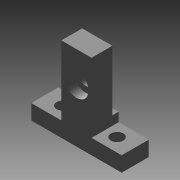
# Autodesk Inventor part: Linear Bearing Adapter Arm
Saved by Autodesk Inventor 2015 SP1 (Build 190203100, 203)
## iProperties
Created: 2015-05-06
Part Number: Linear Bearing Adapter Arm
Material: Generic
Document SubType Name: Modeling
Designer: Andrew
Density: 1 g/cm^3
Appearance: Default
Author: Andrew
Autodesk Inventor part; units mm, degrees
ref_plane "YZ Plane" through (0, 0, 0) normal (1, 0, 0) x (0, 1, 0)
ref_plane "XZ Plane" through (0, 0, 0) normal (0, 1, 0) x (-1, 0, 0)
ref_plane "XY Plane" through (0, 0, 0) normal (0, 0, 1) x (1, 0, 0)
sketch "Sketch1" plane through (0, 0, 0) normal (0, 0, 1) x (1, 0, 0)
  line L0 (15, 0) -> (-15, 0)
  line L1 (-15, 0) -> (-15, 9)
  line L2 (-15, 9) -> (15, 9)
  line L3 (15, 9) -> (15, 0)
  line L4 (0, 10.8) -> (0, -1.8) projected
  circle A0 centre (9, 4.5) radius 2.0625
  circle A1 centre (-9, 4.5) radius 2.0625
  point P0 (0, 0)
  dimension "d0" = 9
  dimension "d1" = 30
  dimension "d4" = 4.125
  dimension "d5" = 6
  dimension "d6" = 4.5
  constraints: 8 end point, 2 centre point, 2 parallel, 1 equal radius, 1 horizontal, 1 midpoint, 1 perpendicular, 2 other
  measures "d0" distance of L0.end L1.end
  measures "d1" distance of L0.start L0.end
  measures "d4" diameter of A0
  measures "d5" distance from line of L3 A0.centre
  measures "d6" distance from line of L0 A0.centre
extrude "Extrusion1" add sketch "Sketch1" along normal blind 5
sketch "Sketch2" plane through (0, 0, 5) normal (0, 0, 1) x (1, 0, 0)
  line L0 (-15, 0) -> (15, 0) projected
  line L1 (15, 9) -> (-15, 9) projected
  line L2 (5, 0) -> (-5, 0)
  line L3 (-5, 0) -> (-5, 9)
  line L4 (-5, 9) -> (5, 9)
  line L5 (5, 9) -> (5, 0)
  line L6 (0, 10.8) -> (0, -1.8) projected
  point P0 (0, 0)
  dimension "d7" = 10
  constraints: 8 end point, 2 parallel, 2 point on line, 1 horizontal, 1 perpendicular, 1 other
  measures "d7" distance between parallel lines of L5 L3
extrude "Extrusion2" add sketch "Sketch2" along normal blind 3
sketch "Sketch3" plane through (0, 0, 8) normal (0, 0, 1) x (1, 0, 0)
  line L0 (-5, 9) -> (-5, 0) projected
  line L1 (5, 0) -> (-5, 0)
  line L2 (-5, 0) -> (-5, 6.9)
  line L3 (-5, 6.9) -> (5, 6.9)
  line L4 (5, 6.9) -> (5, 0)
  point P0 (0, 0)
  dimension "d10" = 6.9
  constraints: 8 end point, 2 parallel, 1 horizontal, 1 perpendicular, 1 point on line
  measures "d10" distance between parallel lines of L1 L3
extrude "Extrusion3" add sketch "Sketch3" along normal blind 20
sketch "Sketch4" plane through (-15, 0, 0) normal (0, -1, 0) x (1, 0, 0)
  circle A0 centre (15, 18) radius 4
  circle A1 centre (15, 18) radius 2.0625
  line L0 (10, 28) -> (20, 28) projected
  point P0 (15, 0)
  dimension "d13" = 8
  dimension "d14" = 4.125
  dimension "d19" = 10
  constraints: 2 centre point, 1 coincident
  measures "d13" diameter of A0
  measures "d14" diameter of A1
  measures "d19" distance from line of L0 A0.centre
extrude "Extrusion4" cut sketch "Sketch4" against normal blind 3 contours A0 | A1
extrude "Extrusion5" cut sketch "Sketch4" against normal up to next contours A1
body "Solid1"
